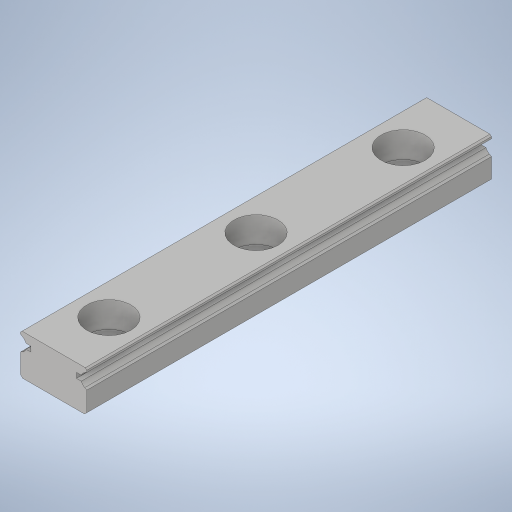
# Autodesk Inventor part: SSEBZ-MX10-55_r
Saved by Autodesk Inventor 2024.1 (Build 281209000, 209)
## iProperties
Category: PARTsolutions
Company: MISUMI
Created: 2022-11-22
Part Number: SSEBZ-MX10-55_r
Material: Generic
Catalog Web Link: www.cadenas.de
Description: SSEBZ, SSEBZ-MX, SSE2BZ, SSE2BZ-MX, SSEBLZ, SSEBLZ-MX, SSE2BLZ, SSE2BLZ-MX, SEBZ, SE2BZ, SEBLZ, SE2BLZ_rail-Miniature Linear Guides - Standard Blocks - Light Preload/Slight Clearance - Standard Grade - Selectable/Configurable
Vendor: MISUMI
Document SubType Name: Modeling
Designer: psAdmin
Manufacturer: MISUMI
Mass: 2.18193 g
Surface Area: 20.8206 cm^2
Volume: 2.18193 cm^3
Density: 1 g/cm^3
Appearance: PSOLRGB-175-175-175
PSOL_IDENT_0: {$CADENAS_DATA/23d-libs/misumi/metric/06_linear_guides/ssebz_series/sebz_rail.prj},303 {VTYP=3D},{NB=
PSOL_IDENT_1: SSEBZ-MX10-55_r},{LINA=SSEBZ-MX10-55},{NN=SSEBZ, SSEBZ-MX, SSE2BZ, SSE2BZ-MX, SSEBLZ, SSEBLZ-MX, SSE
PSOL_IDENT_2: 2BLZ, SSE2BLZ-MX, SEBZ, SE2BZ, SEBLZ, SE2BLZ_rail},{DATE=17.02.2022 00:39:33},{GEOMDATE=20.01.2022 0
PSOL_IDENT_3: 8:28:16},{VERSION=},{LINEID=160},{WBVAR=MAT,MX,NOB,LT,LS,ALT1,ALT2,ALT4},{WBNUMERIC=LS}  {NB=SSEBZ-M
PSOL_IDENT_4: X10-55_r},{LINA=SSEBZ-MX10-55},{KT=DUMMY},{PN=SSEBZ-MX10-55},{RT=B},{TS=Z},{TYPE=SSEBZ},{MAT=S},{MXA
PSOL_IDENT_5: LG='', 'w/o MX(Lubrication unit)', '-MX', 'with MX(Lubrication unit)'},{MX=-MX},{NOB=},{H=10},{LT=Se
PSOL_IDENT_6: lectable},{LTALG='Selectable','Selectable','Configurable','Configurable'},{LS=55},{W=20},{L1=30.0},{
PSOL_IDENT_7: B=15},{C=10},{S=M3x3},{L2=19.0},{K=7.8},{CBB=0.3},{W1=9},{W2=5.5},{H1=5.5},{CAA=0.3},{DD1DD2HH=3.5x6
PSOL_IDENT_8: x3.5},{F=20},{G=7.5},{DD2=6.000},{HH=3.500},{DD1=3.500},{ALT1=},{MC=M4},{MC1=4},{ALT2=},{ALT2L=2.5},
PSOL_IDENT_9: {ALT2N=5},{M=3},{LL=},{L0=35,55,75,95,115,135,155,175,195,215,235,255,275,295,315,335,355,355,375,39
PSOL_IDENT_10: 5,415,435,455,475,495,515,535,555,575,595,615,635},{REC1=   '','w/o Rail Ends Cut alteration','-LLC'
PSOL_IDENT_11: ,'with LLC (Left End Cut)','-RLC','with RLC (Right End Cut)','-LLC-RLC','with Both End Cut'   },{MAT
PSOL_IDENT_12: 2='','Carbon Steel','S','Stainless Steel'},{NL=0.000},{ALT4=},{ALT4ALG= '','Not applicable' },{CA1=0
PSOL_IDENT_13: .2},{CA2=0.3},{VA1=1.5},{HA1=1.4},{HA2=9.5430},{WA1=2.0868},{WA2=0.7},{RA1=2.20},{POIA1=0.1400},{NA1=
PSOL_IDENT_14: 2}
NB: SSEBZ-MX10-55_r
NN: SSEBZ, SSEBZ-MX, SSE2BZ, SSE2BZ-MX, SSEBLZ, SSEBLZ-MX, SSE2BLZ, SSE2BLZ-MX, SEBZ, SE2BZ, SEBLZ, SE2BLZ_rail
NT: Miniature Linear Guides - Standard Blocks - Light Preload/Slight Clearance - Standard Grade - Selectable/Configurable
NBSYN: $PN._r
LINA: SSEBZ-MX10-55
CATALOG: Misumi
PN: SSEBZ-MX10-55
MAT: Stainless Steel
MX: with MX(Lubrication unit)
NOB: 1
H: 10
LT: Selectable
LS: 55
W: 20
L1: 30
B: 15
C: 10
S: M3x3
L2: 19
K: 7.8
CBB: 0.3
W1: 9
W2: 5.5
H1: 5.5
CAA: 0.3
DD1DD2HH: 3.5x6x3.5
F: 20
G: 7.5
ALT1: w/o MC (Tapped Holes)
ALT2: w/o Rail Ends Cut alteration
ALT4: Not applicable
SUPPLIER: MISUMI
ARTICLENO: SSEBZ-MX10-55_r
BOMINFO: SSEBZ-MX10-55
CREATOR: CADENAS GmbH
Title: SSEBZ-MX10-55
Author: Cadenas PARTsolutions
Comments: Miniature Linear Guides - Standard Blocks - Light Preload/Slight Clearance - Standard Grade - Selectable/Configurable
Autodesk Inventor part; units mm, degrees
sketch "Sketch_12" plane through (0, 0, 0) normal (0, 0, 1) x (1, 0, 0)
  line L0 (-4.5, 5.3) -> (-4.5, 5.0434)
  line L1 (-4.5, 5.0434) -> (-4.2216, 4.8827)
  arc A0 (-3.7548, 4.35) -> (-4.2216, 4.8827) centre (-4.7715, 3.93) ccw
  line L2 (-3.7548, 4.35) -> (-3.1, 4.35)
  line L3 (-3.1, 4.35) -> (-3.1, 3.65)
  line L4 (-3.1, 3.65) -> (-3.7548, 3.65)
  arc A1 (-4.2216, 3.1173) -> (-3.7548, 3.65) centre (-4.7715, 4.07) ccw
  line L5 (-4.2216, 3.1173) -> (-4.5, 2.9566)
  line L6 (-4.5, 2.9566) -> (-4.5, 0.3)
  line L7 (-4.5, 0.3) -> (-4.2, 0)
  line L8 (-4.2, 0) -> (4.2, 0)
  line L9 (4.2, 0) -> (4.5, 0.3)
  line L10 (4.5, 0.3) -> (4.5, 2.9566)
  line L11 (4.5, 2.9566) -> (4.2216, 3.1173)
  arc A2 (3.7548, 3.65) -> (4.2216, 3.1173) centre (4.7715, 4.07) ccw
  line L12 (3.7548, 3.65) -> (3.1, 3.65)
  line L13 (3.1, 3.65) -> (3.1, 4.35)
  line L14 (3.1, 4.35) -> (3.7548, 4.35)
  arc A3 (4.2216, 4.8827) -> (3.7548, 4.35) centre (4.7715, 3.93) ccw
  line L15 (4.2216, 4.8827) -> (4.5, 5.0434)
  line L16 (4.5, 5.0434) -> (4.5, 5.3)
  line L17 (4.5, 5.3) -> (4.3, 5.5)
  line L18 (4.3, 5.5) -> (-4.3, 5.5)
  line L19 (-4.3, 5.5) -> (-4.5, 5.3)
  constraints: 40 end point, 8 point on circle, 4 centre point
extrude "Extrusion1" add sketch "Sketch_12" along normal mid plane 55
sketch "Sketch2" plane through (-4.3, 5.5, 27.5) normal (0, 1, 0) x (1, 0, 0)
  point P0 (4.3, 47.5)
hole "Hole1" at (0, 5.5, -20) direction (0, -1, 0) diameter 3.5 depth 5.5 counterbore diameter 6 counterbore depth 3.5
pattern_linear "Rectangular Pattern1" count 3 spacing 20 along (0, 0, 1) of "Hole1"
ref_plane "to_block_XY" through (0, 5.5, 0) normal (0, 0, 1) x (1, 0, 0)
ref_plane "to_block_YZ" through (0, 5.5, 0) normal (1, 0, 0) x (0, 1, 0)
ref_plane "to_block_ZX" through (0, 5.5, 0) normal (0, 1, 0) x (0, 0, 1)
body "Solid1"
